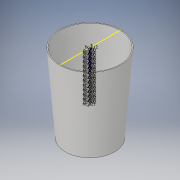
# Autodesk Inventor part: trash bin 13 inches
Saved by Autodesk Inventor 2017 (Build 210142000, 142)
## iProperties
Created: 2018-03-22
Part Number: trash bin 13 inches
Material: Generic
Document SubType Name: Modeling
Designer: Braxton
Density: 1 g/cm^3
Appearance: Default
Author: Braxton
Autodesk Inventor part; units mm, degrees
ref_plane "YZ Plane" through (0, 0, 0) normal (1, 0, 0) x (0, 1, 0)
ref_plane "XZ Plane" through (0, 0, 0) normal (0, 1, 0) x (-1, 0, 0)
ref_plane "XY Plane" through (0, 0, 0) normal (0, 0, 1) x (1, 0, 0)
sketch "Sketch1" plane through (0, 0, 0) normal (0, 0, 1) x (1, 0, 0)
  line L0 (0, 0) -> (0, 27.5167) construction
  line L1 (0, 0) -> (8.4667, 0)
  line L2 (8.4667, 0) -> (10.5833, 27.5167)
  line L3 (10.5833, 27.5167) -> (0, 27.5167) construction
  line L4 (10.5833, 27.5167) -> (10.8871, 27.5167)
  line L5 (10.8871, 27.5167) -> (8.747, -0.3037)
  line L6 (0, -0.3037) -> (8.747, -0.3037)
  line L7 (0, 0) -> (0, -0.3037)
  dimension "d0" = 27.5167
  dimension "d1" = 8.4667
  dimension "d2" = 10.5833
  dimension "d3" = 0.3037
  dimension "d4" = 0.3037
  constraints: 16 end point, 3 parallel, 2 vertical, 1 horizontal, 1 perpendicular
  measures "d0" distance of L0.start L0.end
  measures "d1" distance of L0.start L1.end
  measures "d2" distance of L2.end L0.end
  measures "d3" distance of L2.end L4.end
  measures "d4" distance between parallel lines of L1 L6
revolve "Revolution1" add sketch "Sketch1" angle 360 about axis through (0, 0, 0) along (0, 1, 0)
sketch "Sketch2" plane through (0, 0, 0) normal (1, 0, 0) x (0, 1, 0)
  line L0 (27.0602, 0.0564) -> (27.2129, -0.2082)
  line L1 (27.2129, -0.2082) -> (27.0602, -0.4728)
  line L2 (27.0602, -0.4728) -> (26.7547, -0.4728)
  line L3 (26.7547, -0.4728) -> (26.6019, -0.2082)
  line L4 (26.6019, -0.2082) -> (26.7547, 0.0564)
  line L5 (26.7547, 0.0564) -> (27.0602, 0.0564)
  line L6 (27.5167, 10.8871) -> (27.5167, -10.8871) projected
  line L7 (26.0333, -0.0564) -> (25.8806, 0.2082)
  line L8 (25.8806, 0.2082) -> (26.0333, 0.4728)
  line L9 (26.0333, 0.4728) -> (26.3388, 0.4728)
  line L10 (26.3388, 0.4728) -> (26.4916, 0.2082)
  line L11 (26.4916, 0.2082) -> (26.3388, -0.0564)
  line L12 (26.3388, -0.0564) -> (26.0333, -0.0564)
  line L13 (26.9074, -0.2082) -> (26.1861, 0.2082) construction
  line L14 (27.5167, 0) -> (0, 0)
  line L15 (0, 8.4667) -> (0, -8.4667) projected
  line L16 (25.6175, 0.0564) -> (25.7703, -0.2082)
  line L17 (25.7703, -0.2082) -> (25.6175, -0.4728)
  line L18 (25.6175, -0.4728) -> (25.312, -0.4728)
  line L19 (25.312, -0.4728) -> (25.1593, -0.2082)
  line L20 (25.1593, -0.2082) -> (25.312, 0.0564)
  line L21 (25.312, 0.0564) -> (25.6175, 0.0564)
  line L22 (24.5907, -0.0564) -> (24.4379, 0.2082)
  line L23 (24.4379, 0.2082) -> (24.5907, 0.4728)
  line L24 (24.5907, 0.4728) -> (24.8962, 0.4728)
  line L25 (24.8962, 0.4728) -> (25.049, 0.2082)
  line L26 (25.049, 0.2082) -> (24.8962, -0.0564)
  line L27 (24.8962, -0.0564) -> (24.5907, -0.0564)
  line L28 (25.4648, -0.2082) -> (24.7435, 0.2082) construction
  line L29 (24.1749, 0.0564) -> (24.3276, -0.2082)
  line L30 (24.3276, -0.2082) -> (24.1749, -0.4728)
  line L31 (24.1749, -0.4728) -> (23.8694, -0.4728)
  line L32 (23.8694, -0.4728) -> (23.7166, -0.2082)
  line L33 (23.7166, -0.2082) -> (23.8694, 0.0564)
  line L34 (23.8694, 0.0564) -> (24.1749, 0.0564)
  line L35 (23.1481, -0.0564) -> (22.9953, 0.2082)
  line L36 (22.9953, 0.2082) -> (23.1481, 0.4728)
  line L37 (23.1481, 0.4728) -> (23.4536, 0.4728)
  line L38 (23.4536, 0.4728) -> (23.6063, 0.2082)
  line L39 (23.6063, 0.2082) -> (23.4536, -0.0564)
  line L40 (23.4536, -0.0564) -> (23.1481, -0.0564)
  line L41 (24.0221, -0.2082) -> (23.3008, 0.2082) construction
  line L42 (21.7054, 0.4728) -> (22.0109, 0.4728)
  line L43 (22.0109, 0.4728) -> (22.1637, 0.2082)
  line L44 (21.5527, 0.2082) -> (21.7054, 0.4728)
  line L45 (22.4267, 0.0564) -> (22.7322, 0.0564)
  line L46 (22.1637, 0.2082) -> (22.0109, -0.0564)
  line L47 (22.0109, -0.0564) -> (21.7054, -0.0564)
  line L48 (21.7054, -0.0564) -> (21.5527, 0.2082)
  line L49 (22.274, -0.2082) -> (22.4267, 0.0564)
  line L50 (22.5795, -0.2082) -> (21.8582, 0.2082) construction
  line L51 (22.7322, -0.4728) -> (22.4267, -0.4728)
  line L52 (22.4267, -0.4728) -> (22.274, -0.2082)
  line L53 (22.885, -0.2082) -> (22.7322, -0.4728)
  line L54 (22.7322, 0.0564) -> (22.885, -0.2082)
  line L55 (21.2896, 0.0564) -> (21.4424, -0.2082)
  line L56 (21.4424, -0.2082) -> (21.2896, -0.4728)
  line L57 (21.2896, -0.4728) -> (20.9841, -0.4728)
  line L58 (20.9841, -0.4728) -> (20.8313, -0.2082)
  line L59 (20.8313, -0.2082) -> (20.9841, 0.0564)
  line L60 (20.9841, 0.0564) -> (21.2896, 0.0564)
  line L61 (20.2628, -0.0564) -> (20.11, 0.2082)
  line L62 (20.11, 0.2082) -> (20.2628, 0.4728)
  line L63 (20.2628, 0.4728) -> (20.5683, 0.4728)
  line L64 (20.5683, 0.4728) -> (20.721, 0.2082)
  line L65 (20.721, 0.2082) -> (20.5683, -0.0564)
  line L66 (20.5683, -0.0564) -> (20.2628, -0.0564)
  line L67 (21.1369, -0.2082) -> (20.4155, 0.2082) construction
  line L68 (18.8201, 0.4728) -> (19.1257, 0.4728)
  line L69 (19.1257, 0.4728) -> (19.2784, 0.2082)
  line L70 (18.6674, 0.2082) -> (18.8201, 0.4728)
  line L71 (19.5415, 0.0564) -> (19.847, 0.0564)
  line L72 (19.2784, 0.2082) -> (19.1257, -0.0564)
  line L73 (19.1257, -0.0564) -> (18.8201, -0.0564)
  line L74 (18.8201, -0.0564) -> (18.6674, 0.2082)
  line L75 (19.3887, -0.2082) -> (19.5415, 0.0564)
  line L76 (19.6942, -0.2082) -> (18.9729, 0.2082) construction
  line L77 (19.847, -0.4728) -> (19.5415, -0.4728)
  line L78 (19.5415, -0.4728) -> (19.3887, -0.2082)
  line L79 (19.9997, -0.2082) -> (19.847, -0.4728)
  line L80 (19.847, 0.0564) -> (19.9997, -0.2082)
  line L81 (18.0988, -0.4728) -> (17.9461, -0.2082)
  line L82 (18.0988, 0.0564) -> (18.4043, 0.0564)
  line L83 (18.4043, 0.0564) -> (18.5571, -0.2082)
  line L84 (18.5571, -0.2082) -> (18.4043, -0.4728)
  line L85 (16.9617, 0.0564) -> (17.1144, -0.2082)
  line L86 (17.3775, -0.0564) -> (17.2247, 0.2082)
  line L87 (17.1144, -0.2082) -> (16.9617, -0.4728)
  line L88 (16.6562, 0.0564) -> (16.9617, 0.0564)
  line L89 (17.2247, 0.2082) -> (17.3775, 0.4728)
  line L90 (16.9617, -0.4728) -> (16.6562, -0.4728)
  line L91 (16.3931, 0.2082) -> (16.2404, -0.0564)
  line L92 (16.2404, 0.4728) -> (16.3931, 0.2082)
  line L93 (16.8089, -0.2082) -> (16.0876, 0.2082) construction
  line L94 (16.2404, -0.0564) -> (15.9349, -0.0564)
  line L95 (15.9349, 0.4728) -> (16.2404, 0.4728)
  line L96 (15.7821, 0.2082) -> (15.9349, 0.4728)
  line L97 (15.9349, -0.0564) -> (15.7821, 0.2082)
  line L98 (16.6562, -0.4728) -> (16.5034, -0.2082)
  line L99 (17.9461, -0.2082) -> (18.0988, 0.0564)
  line L100 (17.683, -0.0564) -> (17.3775, -0.0564)
  line L101 (17.3775, 0.4728) -> (17.683, 0.4728)
  line L102 (17.8358, 0.2082) -> (17.683, -0.0564)
  line L103 (18.2516, -0.2082) -> (17.5303, 0.2082) construction
  line L104 (17.683, 0.4728) -> (17.8358, 0.2082)
  line L105 (18.4043, -0.4728) -> (18.0988, -0.4728)
  line L106 (16.5034, -0.2082) -> (16.6562, 0.0564)
  line L107 (15.5191, 0.0564) -> (15.6718, -0.2082)
  line L108 (15.6718, -0.2082) -> (15.5191, -0.4728)
  line L109 (15.5191, -0.4728) -> (15.2135, -0.4728)
  line L110 (15.2135, -0.4728) -> (15.0608, -0.2082)
  line L111 (15.0608, -0.2082) -> (15.2135, 0.0564)
  line L112 (15.2135, 0.0564) -> (15.5191, 0.0564)
  line L113 (14.4922, -0.0564) -> (14.3395, 0.2082)
  line L114 (14.3395, 0.2082) -> (14.4922, 0.4728)
  line L115 (14.4922, 0.4728) -> (14.7977, 0.4728)
  line L116 (14.7977, 0.4728) -> (14.9505, 0.2082)
  line L117 (14.9505, 0.2082) -> (14.7977, -0.0564)
  line L118 (14.7977, -0.0564) -> (14.4922, -0.0564)
  line L119 (15.3663, -0.2082) -> (14.645, 0.2082) construction
  line L120 (13.0496, 0.4728) -> (13.3551, 0.4728)
  line L121 (13.3551, 0.4728) -> (13.5078, 0.2082)
  line L122 (12.8968, 0.2082) -> (13.0496, 0.4728)
  line L123 (13.7709, 0.0564) -> (14.0764, 0.0564)
  line L124 (13.5078, 0.2082) -> (13.3551, -0.0564)
  line L125 (13.3551, -0.0564) -> (13.0496, -0.0564)
  line L126 (13.0496, -0.0564) -> (12.8968, 0.2082)
  line L127 (13.6181, -0.2082) -> (13.7709, 0.0564)
  line L128 (13.9237, -0.2082) -> (13.2023, 0.2082) construction
  line L129 (14.0764, -0.4728) -> (13.7709, -0.4728)
  line L130 (13.7709, -0.4728) -> (13.6181, -0.2082)
  line L131 (14.2292, -0.2082) -> (14.0764, -0.4728)
  line L132 (14.0764, 0.0564) -> (14.2292, -0.2082)
  line L133 (12.3283, -0.4728) -> (12.1755, -0.2082)
  line L134 (12.3283, 0.0564) -> (12.6338, 0.0564)
  line L135 (12.6338, 0.0564) -> (12.7865, -0.2082)
  line L136 (12.7865, -0.2082) -> (12.6338, -0.4728)
  line L137 (11.1911, 0.0564) -> (11.3439, -0.2082)
  line L138 (11.6069, -0.0564) -> (11.4542, 0.2082)
  line L139 (11.3439, -0.2082) -> (11.1911, -0.4728)
  line L140 (10.8856, 0.0564) -> (11.1911, 0.0564)
  line L141 (11.4542, 0.2082) -> (11.6069, 0.4728)
  line L142 (11.1911, -0.4728) -> (10.8856, -0.4728)
  line L143 (10.6226, 0.2082) -> (10.4698, -0.0564)
  line L144 (10.4698, 0.4728) -> (10.6226, 0.2082)
  line L145 (11.0384, -0.2082) -> (10.3171, 0.2082) construction
  line L146 (10.4698, -0.0564) -> (10.1643, -0.0564)
  line L147 (10.1643, 0.4728) -> (10.4698, 0.4728)
  line L148 (10.0115, 0.2082) -> (10.1643, 0.4728)
  line L149 (10.1643, -0.0564) -> (10.0115, 0.2082)
  line L150 (10.8856, -0.4728) -> (10.7329, -0.2082)
  line L151 (12.1755, -0.2082) -> (12.3283, 0.0564)
  line L152 (11.9125, -0.0564) -> (11.6069, -0.0564)
  line L153 (11.6069, 0.4728) -> (11.9125, 0.4728)
  line L154 (12.0652, 0.2082) -> (11.9125, -0.0564)
  line L155 (12.481, -0.2082) -> (11.7597, 0.2082) construction
  line L156 (11.9125, 0.4728) -> (12.0652, 0.2082)
  line L157 (12.6338, -0.4728) -> (12.3283, -0.4728)
  line L158 (10.7329, -0.2082) -> (10.8856, 0.0564)
  point P0 (26.5468, 0)
  point P1 (25.1041, 0)
  point P2 (23.6615, 0)
  point P3 (22.2188, 0)
  point P4 (20.7762, 0)
  point P5 (19.3336, 0)
  point P6 (16.4483, 0)
  point P7 (17.8909, 0)
  point P8 (15.0056, 0)
  point P9 (29.1042, 1.5875)
  point P10 (13.563, 0)
  point P11 (10.6777, 0)
  point P12 (12.1204, 0)
  dimension "d6" = 0.5292
  dimension "d8" = 0.5292
  dimension "d11" = 0.3037
  dimension "d12" = 0.3037
  dimension "d23" = 0.5292
  dimension "d24" = 0.5292
  dimension "d25" = 0.3037
  dimension "d27" = 0.3037
  dimension "d28" = 0.5292
  dimension "d29" = 0.5292
  dimension "d30" = 0.3037
  dimension "d31" = 0.5292
  dimension "d32" = 0.5292
  dimension "d33" = 0.3037
  dimension "d34" = 0.3037
  dimension "d37" = 0.3037
  dimension "d38" = 0.5292
  dimension "d39" = 0.5292
  dimension "d40" = 0.3037
  dimension "d41" = 0.5292
  dimension "d42" = 0.5292
  dimension "d43" = 0.3037
  dimension "d44" = 0.3037
  dimension "d45" = 0.5292
  dimension "d46" = 0.5292
  dimension "d47" = 0.3037
  dimension "d48" = 0.5292
  dimension "d49" = 0.5292
  dimension "d50" = 0.3037
  dimension "d51" = 0.3037
  dimension "d52" = 0.3037
  dimension "d57" = 0.3037
  dimension "d58" = 0.5292
  dimension "d59" = 0.5292
  dimension "d60" = 0.3037
  dimension "d61" = 0.5292
  dimension "d62" = 0.5292
  dimension "d63" = 0.3037
  dimension "d64" = 0.3037
  dimension "d65" = 0.5292
  dimension "d66" = 0.5292
  dimension "d67" = 0.3037
  dimension "d68" = 0.5292
  dimension "d69" = 0.5292
  dimension "d70" = 0.3037
  dimension "d71" = 0.3037
  dimension "d72" = 0.3037
  dimension "d97" = 0.3037
  constraints: 312 end point, 13 midpoint, 12 horizontal, 12 parallel, 12 perpendicular, 1 vertical, 327 other
  measures "d6" distance between parallel lines of L3 L0
  measures "d8" distance between parallel lines of L8 L11
  measures "d11" distance between parallel lines of L11 L4
  measures "d12" distance from line of L6 L0.end
  measures "d23" distance between parallel lines of L19 L16
  measures "d24" distance between parallel lines of L23 L26
  measures "d25" distance between parallel lines of L26 L20
  measures "d27" distance between parallel lines of L7 L16
  measures "d28" distance between parallel lines of L32 L29
  measures "d29" distance between parallel lines of L36 L39
  measures "d30" distance between parallel lines of L39 L33
  measures "d31" distance between parallel lines of L52 L54
  measures "d32" distance between parallel lines of L44 L46
  measures "d33" distance between parallel lines of L46 L49
  measures "d34" distance between parallel lines of L35 L54
  measures "d37" distance between parallel lines of L22 L29
  measures "d38" distance between parallel lines of L58 L55
  measures "d39" distance between parallel lines of L62 L65
  measures "d40" distance between parallel lines of L65 L59
  measures "d41" distance between parallel lines of L78 L80
  measures "d42" distance between parallel lines of L70 L72
  measures "d43" distance between parallel lines of L72 L75
  measures "d44" distance between parallel lines of L61 L80
  measures "d45" distance between parallel lines of L81 L83
  measures "d46" distance between parallel lines of L89 L102
  measures "d47" distance between parallel lines of L102 L99
  measures "d48" distance between parallel lines of L98 L85
  measures "d49" distance between parallel lines of L96 L91
  measures "d50" distance between parallel lines of L91 L106
  measures "d51" distance between parallel lines of L86 L85
  measures "d52" distance between parallel lines of L74 L83
  measures "d57" distance between parallel lines of L48 L55
  measures "d58" distance between parallel lines of L110 L107
  measures "d59" distance between parallel lines of L114 L117
  measures "d60" distance between parallel lines of L117 L111
  measures "d61" distance between parallel lines of L130 L132
  measures "d62" distance between parallel lines of L122 L124
  measures "d63" distance between parallel lines of L124 L127
  measures "d64" distance between parallel lines of L113 L132
  measures "d65" distance between parallel lines of L133 L135
  measures "d66" distance between parallel lines of L141 L154
  measures "d67" distance between parallel lines of L154 L151
  measures "d68" distance between parallel lines of L150 L137
  measures "d69" distance between parallel lines of L148 L143
  measures "d70" distance between parallel lines of L143 L158
  measures "d71" distance between parallel lines of L138 L137
  measures "d72" distance between parallel lines of L126 L135
  measures "d97" distance between parallel lines of L97 L107
equation "\"d4\" = d3"
equation "\"d8\" = d6"
equation "\"d11\" = d3"
equation "\"d12\" = d3"
equation "\"d24\" = d23"
equation "\"d25\" = d26"
equation "\"d27\" = d3"
equation "\"d29\" = d28"
equation "\"d30\" = d35"
equation "\"d32\" = d31"
equation "\"d33\" = d36"
equation "\"d34\" = d35"
equation "\"d37\" = d3"
equation "\"d39\" = d38"
equation "\"d40\" = d53"
equation "\"d42\" = d41"
equation "\"d43\" = d54"
equation "\"d44\" = d53"
equation "\"d46\" = d45"
equation "\"d47\" = d55"
equation "\"d49\" = d48"
equation "\"d50\" = d56"
equation "\"d51\" = d55"
equation "\"d52\" = d53"
equation "\"d57\" = d3"
equation "\"d59\" = d58"
equation "\"d60\" = d89"
equation "\"d62\" = d61"
equation "\"d63\" = d90"
equation "\"d64\" = d89"
equation "\"d66\" = d65"
equation "\"d67\" = d91"
equation "\"d69\" = d68"
equation "\"d70\" = d92"
equation "\"d71\" = d91"
equation "\"d72\" = d89"
equation "\"d26\" = 0.303742"
equation "\"d35\" = 0.303742"
equation "\"d36\" = 0.303742"
equation "\"d53\" = 0.303742"
equation "\"d54\" = 0.303742"
equation "\"d55\" = 0.303742"
equation "\"d56\" = 0.303742"
equation "\"d89\" = 0.303742"
equation "\"d90\" = 0.303742"
equation "\"d91\" = 0.303742"
equation "\"d92\" = 0.303742"
body "Solid1"
